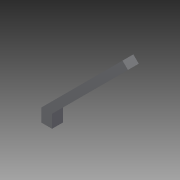
# Autodesk Inventor part: Feeding Mounter
Saved by Autodesk Inventor 2013 (Build 170138000, 138)
## iProperties
Created: 2013-01-26
Part Number: Feeding Mounter
Material: Generic
Document SubType Name: Modeling
Designer: actoennies
Density: 1 g/cm^3
Author: actoennies
Autodesk Inventor part; units mm, degrees
ref_plane "YZ Plane" through (0, 0, 0) normal (1, 0, 0) x (0, 1, 0)
ref_plane "XZ Plane" through (0, 0, 0) normal (0, 1, 0) x (-1, 0, 0)
ref_plane "XY Plane" through (0, 0, 0) normal (0, 0, 1) x (1, 0, 0)
sketch "Sketch1" plane through (0, 0, 0) normal (0, 0, 1) x (1, 0, 0)
  line L0 (0, 0) -> (0, 7.62)
  line L1 (0, 0) -> (6.35, 0)
  line L2 (6.35, 0) -> (6.35, 7.62)
  line L3 (0, 7.62) -> (47.7314, 55.3514)
  line L4 (6.35, 7.62) -> (50.9064, 52.1764)
  line L5 (50.9064, 52.1764) -> (47.7314, 55.3514)
  dimension "d1" = 7.62
  dimension "d2" = 6.35
  dimension "d3" = 7.62
  dimension "d4" = 45
  dimension "d5" = 3.175
  dimension "d6" = 3.175
  constraints: 12 end point, 3 perpendicular, 1 parallel, 1 vertical
  measures "d1" distance of L0.start L0.end
  measures "d2" distance of L0.start L1.end
  measures "d3" distance of L1.end L2.end
  measures "d4" angle of L3 L0
  measures "d5" horizontal distance of L4.end L3.end
  measures "d6" horizontal distance of L4.end L3.end
extrude "Extrusion1" add sketch "Sketch1" along normal blind 6.35
body "Solid1"
